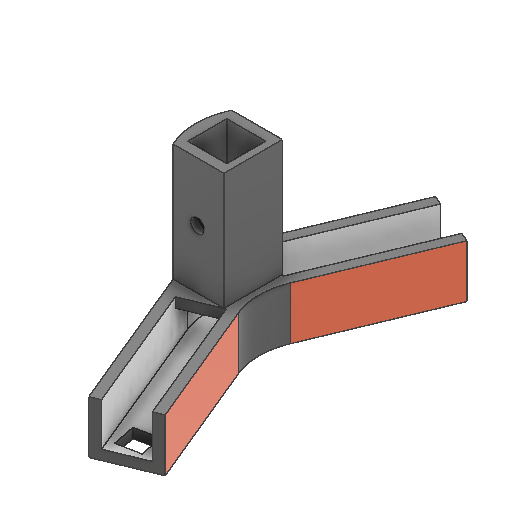
# Autodesk Inventor part: 135FootUpdateWires
Saved by Autodesk Inventor 2025.2 (Build 292293000, 293)
## iProperties
Created: 2024-08-13
Part Number: 135FootUpdateWires
Material: Generic
Document SubType Name: Modeling
Designer: 16366081
Density: 1 g/cm^3
Appearance: Default
Author: 16366081
Autodesk Inventor part; units mm, degrees
ref_plane "YZ Plane" through (0, 0, 0) normal (1, 0, 0) x (0, 1, 0)
ref_plane "XZ Plane" through (0, 0, 0) normal (0, 1, 0) x (-1, 0, 0)
ref_plane "XY Plane" through (0, 0, 0) normal (0, 0, 1) x (1, 0, 0)
sketch "Sketch1" plane through (0, 0, 0) normal (0, 1, 0) x (-1, 0, 0)
  line L0 (-10, 10) -> (10, 10) construction
  line L1 (10, 10) -> (10, -10) construction
  line L2 (10, -10) -> (-10, -10) construction
  line L3 (-10, -10) -> (-10, 10) construction
  line L4 (-10, 10) -> (10, -10) construction
  line L5 (10, 10) -> (-10, -10) construction
  line L6 (0, 0) -> (-34.4415, -83.1492) construction
  line L7 (0, 0) -> (-50, 0) construction
  line L8 (0, 0) -> (-34.4415, 83.1492) construction
  line L9 (-11.1522, -0.7926) -> (7.3254, -8.4462) construction
  line L10 (7.3254, -8.4462) -> (-57.7308, -165.5058) construction
  line L11 (-57.7308, -165.5058) -> (-76.2084, -157.8521) construction
  line L12 (-76.2084, -157.8521) -> (-11.1522, -0.7926) construction
  line L13 (-11.1522, -0.7926) -> (-57.7308, -165.5058) construction
  line L14 (7.3254, -8.4462) -> (-76.2084, -157.8521) construction
  line L15 (-11.1522, 0.7926) -> (7.3254, 8.4462) construction
  line L16 (7.3254, 8.4462) -> (-57.7308, 165.5058) construction
  line L17 (-57.7308, 165.5058) -> (-76.2084, 157.8521) construction
  line L18 (-76.2084, 157.8521) -> (-11.1522, 0.7926) construction
  line L19 (-11.1522, 0.7926) -> (-57.7308, 165.5058) construction
  line L20 (7.3254, 8.4462) -> (-76.2084, 157.8521) construction
  line L21 (-34.4415, -83.1492) -> (-20.5833, -88.8894)
  line L22 (-34.4415, -83.1492) -> (-19.4415, -83.1492) construction
  line L23 (-20.5833, -88.8894) -> (16.2359, 0)
  line L24 (-34.4415, 83.1492) -> (-20.5833, 88.8894)
  line L25 (-34.4415, 83.1492) -> (-19.4415, 83.1492) construction
  line L26 (-20.5833, 88.8894) -> (16.2359, 0)
  line L27 (-34.4415, -83.1492) -> (-48.2997, -77.4089)
  line L28 (-48.2997, -77.4089) -> (-16.2359, 0)
  line L29 (-34.4415, 83.1492) -> (-48.2997, 77.4089)
  line L30 (-34.4415, 83.1492) -> (-19.4415, 83.1492) construction
  line L31 (-48.2997, 77.4089) -> (-16.2359, 0)
  line L32 (0, 0) -> (-30.6147, -73.9104) construction
  dimension "d0" = 20
  dimension "d1" = 20
  dimension "d3" = 50
  dimension "d4" = 90
  dimension "d5" = 90
  dimension "d6" = 67.5
  dimension "d7" = 67.5
  dimension "d10" = 20
  dimension "d11" = 170
  dimension "d12" = 20
  dimension "d13" = 170
  dimension "d14" = 15
  dimension "d15" = 22.5
  dimension "d16" = 15
  dimension "d17" = 22.5
  dimension "d18" = 15
  dimension "d19" = 90
  dimension "d20" = 15
  dimension "d21" = 157.5
  dimension "d90" = 80
  constraints: 66 end point, 9 perpendicular, 6 midpoint, 6 parallel, 5 horizontal, 3 equal length, 1 point on line
  measures "d0" distance of L1.end L2.end
  measures "d1" distance of L0.end L1.end
  measures "d3" distance of L6.start L7.end
  measures "d4" distance of L6.start L6.end
  measures "d5" distance of L6.start L8.end
  measures "d6" angle of L7 L6
  measures "d7" angle of L7 L8
  measures "d10" distance of L9.start L9.end
  measures "d11" distance of L9.end L10.end
  measures "d12" distance of L15.start L15.end
  measures "d13" distance of L16.end L15.end
  measures "d14" distance of L6.end L21.end
  measures "d15" angle of L21 L22
  measures "d16" distance of L8.end L24.end
  measures "d17" angle of L25 L24
  measures "d18" distance of L6.end L27.end
  measures "d19" angle of L27 L28
  measures "d20" distance of L8.end L29.end
  measures "d21" angle of L29 L30
  measures "d90" distance of L6.start L32.end
extrude "Extrusion1" add sketch "Sketch1" along normal blind 24
sketch "Sketch3" plane through (48.2997, 0, 77.4089) normal (0.3826834, 0, 0.9238795) x (0.9238795, 0, -0.3826834)
  line L0 (-25, 2) -> (-5, 2)
  line L1 (-5, 2) -> (-5, 22)
  line L2 (-5, 22) -> (-25, 22)
  line L3 (-25, 22) -> (-25, 2)
  line L4 (-25, 2) -> (-5, 22) construction
  line L5 (-5, 2) -> (-25, 22) construction
  line L6 (-30, 0) -> (0, 0) projected
  point P0 (-15, 0)
  point P1 (-15, 12)
  dimension "d30" = 20
  dimension "d31" = 20
  dimension "d155" = 12
  constraints: 12 end point, 2 midpoint, 2 parallel, 1 horizontal, 1 perpendicular
  measures "d30" distance of L2.end L1.end
  measures "d31" distance of L1.end L0.end
  measures "d155" distance from line of L6 point (-15, 12)
extrude "Extrusion3" cut sketch "Sketch3" against normal blind 70
sketch "Sketch4" plane through (20.5833, 0, -88.8894) normal (0.3826834, 0, -0.9238795) x (-0.9238795, 0, -0.3826834)
  line L0 (-25, 22) -> (-5, 22)
  line L1 (-5, 22) -> (-5, 2)
  line L2 (-5, 2) -> (-25, 2)
  line L3 (-25, 2) -> (-25, 22)
  line L4 (-25, 22) -> (-5, 2) construction
  line L5 (-5, 22) -> (-25, 2) construction
  point P0 (-15, 0)
  point P1 (-15, 12)
  dimension "d34" = 20
  dimension "d35" = 20
  constraints: 12 end point, 2 midpoint, 2 parallel, 1 horizontal, 1 perpendicular
  measures "d34" distance of L1.end L2.end
  measures "d35" distance of L0.end L1.end
extrude "Extrusion4" cut sketch "Sketch4" against normal blind 70
sketch "Sketch7" plane through (0, 24, 0) normal (0, 1, 0) x (1, 0, 0)
  line L0 (16, -15) -> (-11, -15)
  line L1 (-11, -15) -> (-11, 15)
  line L2 (-11, 15) -> (16, 15)
  line L3 (16, 15) -> (16, -15)
  line L4 (16, -15) -> (-11, 15) construction
  line L5 (-11, -15) -> (16, 15) construction
  line L6 (-11, -15) -> (-10.0227, -15)
  line L7 (-16.2359, 0) -> (20.5833, -88.8894) projected
  line L8 (20.5833, 88.8894) -> (-16.2359, 0) projected
  line L9 (-16.2359, 0) -> (-10.0227, 15)
  line L10 (-10.0227, 15) -> (-11, 15)
  line L11 (16, -15) -> (22.4491, -15)
  line L12 (48.2997, -77.4089) -> (16.2359, 0) projected
  line L13 (16, 15) -> (20.4136, 15)
  line L14 (22.4491, -15) -> (16.2359, 0)
  line L15 (16.2359, 0) -> (48.2997, 77.4089) projected
  line L16 (16.2359, 0) -> (22.4491, -15)
  point P0 (0, 0)
  point P1 (2.5, 0)
  point P2 (-11, 12.6405)
  point P3 (-11, -12.6405)
  point P4 (-10.0227, -15)
  dimension "d48" = 27
  dimension "d49" = 30
  dimension "d50" = 2.5
  constraints: 26 end point, 4 horizontal, 3 parallel, 3 point on line, 2 collinear, 2 midpoint, 1 horizontal alignment, 1 perpendicular, 1 other
  measures "d48" distance of L1.end L2.end
  measures "d49" distance of L0.end L1.end
  measures "d50" distance of point (0, 0) point (2.5, 0)
extrude "Extrusion14" add sketch "Sketch7" along normal blind 60 contours L0 L7 L1 L8 L2 L3 | L7 L8 L1
sketch "Sketch14" plane through (0, 84, 0) normal (0, 1, 0) x (1, 0, 0)
  line L0 (12.5, -10) -> (-7.5, -10)
  line L1 (-7.5, -10) -> (-7.5, 10)
  line L2 (-7.5, 10) -> (12.5, 10)
  line L3 (12.5, 10) -> (12.5, -10)
  line L4 (12.5, -10) -> (-7.5, 10) construction
  line L5 (-7.5, -10) -> (12.5, 10) construction
  point P0 (0, 0)
  point P1 (2.5, 0)
  dimension "d85" = 20
  dimension "d86" = 20
  dimension "d87" = 2.5
  constraints: 12 end point, 2 midpoint, 2 parallel, 1 horizontal, 1 horizontal alignment, 1 perpendicular
  measures "d85" distance of L1.end L2.end
  measures "d86" distance of L0.end L1.end
  measures "d87" distance of point (2.5, 0) point (0, 0)
extrude "Extrusion15" cut sketch "Sketch14" against normal blind 60
sketch "Sketch15" plane through (0, 0, 0) normal (0, -1, 0) x (1, 0, 0)
  line L0 (0, 0) -> (30.6147, -73.9104) construction
  line L1 (48.2997, -77.4089) -> (20.5833, -88.8894) construction
  line L2 (0, 0) -> (80, 0) construction
  line L3 (0, 0) -> (30.6147, 73.9104) construction
  line L4 (16.8925, 14.6508) -> (-1.5851, 22.3044) construction
  line L5 (0, 0) -> (80, 0) construction
  line L6 (30.6147, 73.9104) -> (30.6147, -73.9104) construction
  line L7 (37.6699, -78.6245) -> (25.9005, -80.9656)
  line L8 (25.9005, -80.9656) -> (23.5594, -69.1962)
  line L9 (23.5594, -69.1962) -> (35.3288, -66.8551)
  line L10 (35.3288, -66.8551) -> (37.6699, -78.6245)
  line L11 (37.6699, -78.6245) -> (23.5594, -69.1962) construction
  line L12 (25.9005, -80.9656) -> (35.3288, -66.8551) construction
  line L13 (35.3288, 66.8551) -> (23.5594, 69.1962)
  line L14 (23.5594, 69.1962) -> (25.9005, 80.9656)
  line L15 (25.9005, 80.9656) -> (37.6699, 78.6245)
  line L16 (37.6699, 78.6245) -> (35.3288, 66.8551)
  line L17 (35.3288, 66.8551) -> (25.9005, 80.9656) construction
  line L18 (23.5594, 69.1962) -> (37.6699, 78.6245) construction
  circle A0 centre (15.3073, 36.9552) radius 4
  circle A1 centre (15.3073, -36.9552) radius 4
  line L19 (30.6147, -73.9104) -> (15.3073, -36.9552) construction
  dimension "d91" = 80
  dimension "d92" = 67.5
  dimension "d93" = 80
  dimension "d94" = 67.5
  dimension "d97" = 12
  dimension "d98" = 12
  dimension "d100" = 101.25
  dimension "d101" = 12
  dimension "d102" = 12
  dimension "d103" = 101.25
  dimension "d107" = 8
  dimension "d108" = 8
  dimension "d109" = 40
  dimension "d110" = 40
  constraints: 36 end point, 6 midpoint, 4 parallel, 4 perpendicular, 2 centre point, 2 equal length, 2 horizontal, 1 collinear
  measures "d91" distance of L0.start L0.end
  measures "d92" angle of L0 L2
  measures "d93" distance of L0.start L3.end
  measures "d94" angle of L5 L3
  measures "d97" distance of L8.end L9.end
  measures "d98" distance of L7.end L8.end
  measures "d100" angle of L9 L0
  measures "d101" distance of L14.end L15.end
  measures "d102" distance of L13.end L14.end
  measures "d103" angle of L3 L13
  measures "d107" diameter of A0
  measures "d108" diameter of A1
  measures "d109" distance of L3.end A0.centre
  measures "d110" distance of L0.end L19.end
extrude "Extrusion16" cut sketch "Sketch15" against normal blind 15 contours L7 L8 L9 L10 | L13 L14 L15 L16
fillet "Fillet1" radius 35 2 edges at (16.2359, 12, 0) (-16.2359, 42, 0)
sketch "Sketch26" plane through (0, 24, 0) normal (0, 1, 0) x (1, 0, 0)
  line L0 (25.2027, -86.976) -> (43.6803, -79.3223) projected
  line L1 (-1.5851, -22.3044) -> (16.8925, -14.6508) projected
  line L2 (43.6803, -79.3223) -> (16.8925, -14.6508) projected
  line L3 (25.2027, -86.976) -> (-1.5851, -22.3044) projected
  line L4 (25.2027, -86.976) -> (-4.6107, -15)
  line L5 (16, -15) -> (-10.0227, -15) projected
  line L6 (17.0371, -15) -> (43.6803, -79.3223)
  point P0 (0, 0)
  point P1 (21.4279, -12.5)
  point P2 (-11.0439, -12.5)
  point P3 (9.0192, -12.5)
  point P4 (-10.0227, -15)
  constraints: 4 end point, 2 point on line, 1 perpendicular, 3 other
extrude "Extrusion28" cut sketch "Sketch26" against normal blind 10
sketch "Sketch27" plane through (0, 24, 0) normal (0, 1, 0) x (1, 0, 0)
  line L0 (43.6803, 79.3223) -> (25.2027, 86.976) projected
  line L1 (43.6803, 79.3223) -> (16.8925, 14.6508) projected
  line L2 (16.8925, 14.6508) -> (-1.5851, 22.3044) projected
  line L3 (25.2027, 86.976) -> (-1.5851, 22.3044) projected
  line L4 (43.6803, 79.3223) -> (42.6451, 76.8231)
  line L5 (16.8925, 14.6508) -> (-1.5851, 22.3044) projected
  line L6 (16.8925, 14.6508) -> (-1.5851, 22.3044)
  line L7 (-1.5851, 22.3044) -> (25.2027, 86.976)
  point P0 (0, 0)
  constraints: 6 end point, 1 collinear, 1 perpendicular, 1 point on line
extrude "Extrusion29" cut sketch "Sketch27" against normal blind 10
sketch "Sketch28" plane through (0, 84, 0) normal (0, 1, 0) x (1, 0, 0)
  line L0 (12.5, 10) -> (12.5, -10) projected
  line L1 (12.5, -10) -> (20.5786, -10)
  arc A0 (21.7838, 13.3939) -> (21.7838, -13.3939) centre (54.1196, 0) ccw projected
  arc A1 (-10.6879, 13.3939) -> (-10.6879, -13.3939) centre (21.6478, 0) ccw projected
  line L2 (-10.0227, -15) -> (16, -15) projected
  line L3 (16, 15) -> (-10.0227, 15) projected
  line L4 (-7.5, -10) -> (-7.5, 10) projected
  line L5 (-7.5, 10) -> (12.5, 10) projected
  line L6 (12.5, 10) -> (12.5, -10) projected
  line L7 (12.5, -10) -> (-7.5, -10) projected
  line L8 (12.5, -10) -> (12.5, 10)
  line L9 (20.5786, 10) -> (12.5, 10)
  arc A2 (20.5786, 10) -> (20.5786, -10) centre (54.1196, 0) ccw
  line L10 (16, -15) -> (16, 15) projected
  line L11 (-10.6879, -13.3939) -> (-10.0227, -15) projected
  line L12 (-10.0227, 15) -> (-10.6879, 13.3939) projected
  point P0 (0, 0)
  constraints: 6 end point, 3 point on circle, 1 centre point, 1 collinear, 1 horizontal, 1 perpendicular
extrude "Extrusion30" [suppressed]
sketch "Sketch30" plane through (-10.0227, 24, 15) normal (0, 0, 1) x (1, 0, 0)
  circle A0 centre (12.5227, 30) radius 3.5
  line L0 (26.0227, 0) -> (26.0227, 60) projected
  line L1 (22.5227, 60) -> (2.5227, 60) projected
  line L2 (22.5227, 60) -> (22.5227, 0) projected
  line L3 (22.5227, 0) -> (2.5227, 0) projected
  line L4 (2.5227, 60) -> (2.5227, 0) projected
  point P0 (10.0227, -24)
  point P1 (26.0227, 30)
  point P2 (22.5227, 30)
  point P3 (12.5227, 60)
  dimension "d167" = 7
  dimension "d169" = 10
  dimension "d170" = 30
  constraints: 3 midpoint, 1 centre point
  measures "d167" diameter of A0
  measures "d169" distance of A0.centre point (22.523, 30)
  measures "d170" distance of A0.centre point (12.523, 60)
extrude "Extrusion32" cut sketch "Sketch30" against normal blind 4 contours A0
sketch "Sketch31" plane through (2.5, 54, 11) normal (0, 0, 1) x (1, 0, 0)
  circle A0 centre (0, 0) radius 2
  circle A1 centre (0, 0) radius 3.5 projected
  point P0 (-2.5, -54)
  dimension "d173" = 4
  constraints: 1 centre point, 1 concentric
  measures "d173" diameter of A0
extrude "Extrusion33" cut sketch "Sketch31" against normal through all contours A0
sketch "Sketch32" plane through (16, 24, -15) normal (0, 0, -1) x (-1, 0, 0)
  line L0 (23.5, 60) -> (3.5, 60) projected
  line L1 (23.5, 60) -> (23.5, 0) projected
  line L2 (23.5, 0) -> (3.5, 0) projected
  line L3 (3.5, 60) -> (3.5, 0) projected
  circle A0 centre (13.5, 30) radius 3.5
  line L4 (0, 60) -> (26.0227, 60) projected
  point P0 (16, -24)
  point P1 (13.0113, 60)
  dimension "d176" = 7
  dimension "d177" = 10
  dimension "d178" = 30
  constraints: 1 centre point, 1 midpoint
  measures "d176" diameter of A0
  measures "d177" distance from line of L1 A0.centre
  measures "d178" vertical distance of point (13.011, 60) A0.centre
extrude "Extrusion34" cut sketch "Sketch32" against normal blind 4 contours A0
sketch "Sketch33" plane through (48.2997, 0, 77.4089) normal (0.9238795, 0, -0.3826834) x (-0.3826834, 0, -0.9238795)
  line L0 (70, 24) -> (70, 2) projected
  line L1 (0, 2) -> (70, 2) projected
  line L2 (0, 24) -> (0, 2) projected
  line L3 (70, 24) -> (0, 24) projected
  circle A0 centre (30, 12) radius 3.5
  point P0 (90, 0)
  dimension "d181" = 7
  dimension "d183" = 10
  dimension "d184" = 30
  constraints: 1 centre point
  measures "d181" diameter of A0
  measures "d183" distance from line of L1 A0.centre
  measures "d184" distance from line of A0.centre L2
extrude "Extrusion35" [suppressed]
sketch "Sketch34" plane through (20.5833, 0, 88.8894) normal (-0.9238795, 0, 0.3826834) x (0.3826834, 0, 0.9238795)
  circle A0 centre (-30, 12) radius 3.5
  line L0 (-81.7157, 0) -> (0, 0) projected
  line L1 (0, 2) -> (0, 24) projected
  line L2 (0, 2) -> (-70, 2) projected
  line L3 (-70, 24) -> (-70, 2) projected
  line L4 (0, 24) -> (-70, 24) projected
  point P0 (-90, 0)
  point P1 (0, 13)
  dimension "d187" = 7
  dimension "d188" = 10
  dimension "d189" = 30
  constraints: 1 centre point, 1 midpoint
  measures "d187" diameter of A0
  measures "d188" distance from line of L2 A0.centre
  measures "d189" horizontal distance of point (0, 13) A0.centre
extrude "Extrusion36" [suppressed]
sketch "Sketch35" plane through (33.1237, 12, 51.2233) normal (0.9238795, 0, -0.3826834) x (-0.3826834, 0, -0.9238795)
  circle A0 centre (0, 0) radius 2
  circle A1 centre (0, 0) radius 3.5 projected
  point P0 (60, -12)
  dimension "d192" = 4
  constraints: 1 centre point, 1 concentric
  measures "d192" diameter of A0
extrude "Extrusion37" [suppressed]
sketch "Sketch36" plane through (48.2997, 0, -77.4089) normal (0.9238795, 0, 0.3826834) x (0.3826834, 0, -0.9238795)
  circle A0 centre (-30, 12) radius 3.5
  line L0 (0, 2) -> (0, 24) projected
  line L1 (0, 2) -> (-70, 2) projected
  line L2 (-70, 24) -> (-70, 2) projected
  line L3 (0, 24) -> (-70, 24) projected
  point P0 (-90, 0)
  dimension "d195" = 7
  dimension "d196" = 30
  dimension "d197" = 10
  constraints: 1 centre point
  measures "d195" diameter of A0
  measures "d196" distance from line of L0 A0.centre
  measures "d197" distance from line of L1 A0.centre
extrude "Extrusion38" [suppressed]
sketch "Sketch37" plane through (20.5833, 0, -88.8894) normal (-0.9238795, 0, -0.3826834) x (-0.3826834, 0, 0.9238795)
  circle A0 centre (30, 12) radius 3.5
  line L0 (0, 0) -> (81.7157, 0) projected
  line L1 (70, 24) -> (70, 2) projected
  line L2 (0, 2) -> (70, 2) projected
  line L3 (0, 24) -> (0, 2) projected
  line L4 (70, 24) -> (0, 24) projected
  line L5 (0, 0) -> (0, 24) projected
  point P0 (90, 0)
  point P1 (0, 12)
  dimension "d200" = 7
  dimension "d201" = 10
  dimension "d202" = 30
  constraints: 1 centre point, 1 midpoint
  measures "d200" diameter of A0
  measures "d201" distance from line of L2 A0.centre
  measures "d202" distance of point (0, 12) A0.centre
extrude "Extrusion39" [suppressed]
sketch "Sketch38" plane through (12.7983, 12, -59.6423) normal (-0.9238795, 0, -0.3826834) x (-0.3826834, 0, 0.9238795)
  circle A0 centre (0, 0) radius 2
  circle A1 centre (0, 0) radius 3.5 projected
  point P0 (60, -12)
  dimension "d205" = 4
  constraints: 1 centre point, 1 concentric
  measures "d205" diameter of A0
extrude "Extrusion40" [suppressed]
sketch "Sketch40" plane through (0, 0, 0) normal (0, -1, 0) x (1, 0, 0)
  arc A0 (-10.6879, 13.3939) -> (-10.6879, -13.3939) centre (21.6478, 0) ccw projected
  line L0 (20.5833, -88.8894) -> (-10.6879, -13.3939) projected
  line L1 (48.2997, -77.4089) -> (20.5833, -88.8894) projected
  line L2 (21.7838, -13.3939) -> (48.2997, -77.4089) projected
  arc A1 (21.7838, 13.3939) -> (21.7838, -13.3939) centre (54.1196, 0) ccw projected
  line L3 (48.2997, 77.4089) -> (21.7838, 13.3939) projected
  line L4 (20.5833, 88.8894) -> (48.2997, 77.4089) projected
  line L5 (-10.6879, 13.3939) -> (20.5833, 88.8894) projected
  line L6 (25.9005, -80.9656) -> (23.5594, -69.1962) projected
  line L7 (23.5594, -69.1962) -> (35.3288, -66.8551) projected
  line L8 (35.3288, -66.8551) -> (37.6699, -78.6245) projected
  line L9 (37.6699, -78.6245) -> (25.9005, -80.9656) projected
  line L10 (23.5594, 69.1962) -> (25.9005, 80.9656) projected
  line L11 (25.9005, 80.9656) -> (37.6699, 78.6245) projected
  line L12 (37.6699, 78.6245) -> (35.3288, 66.8551) projected
  line L13 (35.3288, 66.8551) -> (23.5594, 69.1962) projected
  line L14 (20.5833, 88.8894) -> (48.2997, 77.4089) projected
  line L15 (48.2997, 77.4089) -> (20.5833, 88.8894)
  line L16 (20.5833, 88.8894) -> (-10.6879, 13.3939)
  arc A2 (-10.6879, 13.3939) -> (-10.6879, -13.3939) centre (21.6478, 0) ccw projected
  arc A3 (-10.6879, 13.3939) -> (-10.6879, -13.3939) centre (21.6478, 0) ccw
  line L17 (-10.6879, -13.3939) -> (20.5833, -88.8894)
  line L18 (48.2997, -77.4089) -> (21.7838, -13.3939)
  arc A4 (21.7838, 13.3939) -> (21.7838, -13.3939) centre (54.1196, 0) ccw
  arc A5 (21.7838, 13.3939) -> (21.7838, -13.3939) centre (54.1196, 0) ccw projected
  line L19 (48.2997, 77.4089) -> (21.7838, 13.3939) projected
  line L20 (21.7838, 13.3939) -> (48.2997, 77.4089)
  point P0 (0, 0)
  constraints: 10 end point, 5 point on circle, 4 collinear, 2 centre point, 2 concentric, 1 point on line
extrude "Extrusion41" add sketch "Sketch40" along normal blind 3
sketch "Sketch41" plane through (0, -3, 0) normal (0, -1, 0) x (1, 0, 0)
  circle A0 centre (17.2208, -41.5746) radius 3.5
  line L0 (-10.6879, -13.3939) -> (20.5833, -88.8894) projected
  line L1 (20.5833, -88.8894) -> (48.2997, -77.4089) projected
  point P0 (0, 0)
  dimension "d213" = 7
  dimension "d214" = 15
  dimension "d215" = 45
  constraints: 1 centre point
  measures "d213" diameter of A0
  measures "d214" distance from line of L0 A0.centre
  measures "d215" distance from line of L1 A0.centre
extrude "Extrusion42" cut sketch "Sketch41" against normal blind 4
sketch "Sketch42" plane through (17.2208, 1, -41.5746) normal (0, -1, 0) x (1, 0, 0)
  circle A0 centre (0, 0) radius 2
  point P0 (-17.2208, 41.5746)
  dimension "d218" = 4
  constraints: 1 centre point
  measures "d218" diameter of A0
extrude "Extrusion43" cut sketch "Sketch42" against normal through all
mirror "Mirror1" about plane through (0, 0, 0) normal (0, 0, 1) of "Extrusion42", "Extrusion43"
shell "Shell1" thickness 5 removed faces 2 at (10.7325, 15.3333, -17.2001) at (10.7325, 15.3333, 17.2001)
body "Solid1"
